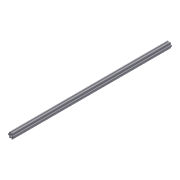
# Autodesk Inventor part: CrossHex 1825
Saved by Autodesk Inventor 2011 (Build 150239000, 239)
## iProperties
Created: 2011-07-24
Part Number: CrossHex 1825
Material: Aluminum-6061
Document SubType Name: Modeling
Designer: Dan Niemitalo
Mass: 103.792 g
Surface Area: 304.789 cm^2
Volume: 38.2997 cm^3
Density: 2.71 g/cm^3
Author: Dan Niemitalo
Autodesk Inventor part; units mm, degrees
ref_plane "YZ Plane" through (0, 0, 0) normal (1, 0, 0) x (0, 1, 0)
ref_plane "XZ Plane" through (0, 0, 0) normal (0, 1, 0) x (-1, 0, 0)
ref_plane "XY Plane" through (0, 0, 0) normal (0, 0, 1) x (1, 0, 0)
sketch "CrossHexProfile" plane through (0, 0, 0) normal (0, 0, 1) x (1, 0, 0)
  arc A0 (1.7598, 0) -> (1.5084, -0.2177) centre (1.7598, -0.254) ccw
  line L0 (1.7598, 0) -> (3.5929, 0)
  arc A1 (3.7028, -0.0635) -> (3.5929, 0) centre (3.5929, -0.127) ccw
  line L1 (3.7028, -0.0635) -> (4.6194, -1.651)
  arc A2 (4.5565, -1.9776) -> (4.6194, -1.651) centre (4.3994, -1.778) ccw
  arc A3 (4.5565, -1.9776) -> (6.0649, -4.5901) centre (5.4993, -3.175) ccw
  arc A4 (-1.5084, -0.2177) -> (1.5084, -0.2177) centre (0, 0) ccw
  arc A5 (-4.5565, -10.7224) -> (-4.6194, -11.049) centre (-4.3994, -10.922) ccw
  arc A6 (-4.5565, -10.7224) -> (-6.0649, -8.1099) centre (-5.4993, -9.525) ccw
  arc A7 (-6.3791, -8.001) -> (-6.0649, -8.1099) centre (-6.1592, -7.874) ccw
  line L2 (-6.3791, -8.001) -> (-7.2957, -6.4135)
  arc A8 (-7.2957, -6.2865) -> (-7.2957, -6.4135) centre (-7.1857, -6.35) ccw
  arc A9 (-6.0649, -4.5901) -> (-6.3791, -4.699) centre (-6.1592, -4.826) ccw
  line L3 (-7.2957, -6.2865) -> (-6.3791, -4.699)
  arc A10 (-1.5084, -0.2177) -> (-1.7598, 0) centre (-1.7598, -0.254) ccw
  line L4 (-3.5929, 0) -> (-1.7598, 0)
  arc A11 (-3.5929, 0) -> (-3.7028, -0.0635) centre (-3.5929, -0.127) ccw
  line L5 (-4.6194, -1.651) -> (-3.7028, -0.0635)
  arc A12 (-4.6194, -1.651) -> (-4.5565, -1.9776) centre (-4.3994, -1.778) ccw
  arc A13 (-6.0649, -4.5901) -> (-4.5565, -1.9776) centre (-5.4993, -3.175) ccw
  line L6 (-3.7028, -12.6365) -> (-4.6194, -11.049)
  circle A14 centre (0, -6.35) radius 2.9337
  arc A15 (-3.7028, -12.6365) -> (-3.5929, -12.7) centre (-3.5929, -12.573) ccw
  line L7 (-1.7598, -12.7) -> (-3.5929, -12.7)
  arc A16 (-1.7598, -12.7) -> (-1.5084, -12.4823) centre (-1.7598, -12.446) ccw
  arc A17 (1.5084, -12.4823) -> (-1.5084, -12.4823) centre (0, -12.7) ccw
  arc A18 (1.5084, -12.4823) -> (1.7598, -12.7) centre (1.7598, -12.446) ccw
  line L8 (3.5929, -12.7) -> (1.7598, -12.7)
  arc A19 (3.5929, -12.7) -> (3.7028, -12.6365) centre (3.5929, -12.573) ccw
  line L9 (4.6194, -11.049) -> (3.7028, -12.6365)
  arc A20 (6.3791, -4.699) -> (6.0649, -4.5901) centre (6.1592, -4.826) ccw
  line L10 (6.3791, -4.699) -> (7.2957, -6.2865)
  arc A21 (7.2957, -6.4135) -> (7.2957, -6.2865) centre (7.1857, -6.35) ccw
  arc A22 (6.0649, -8.1099) -> (6.3791, -8.001) centre (6.1592, -7.874) ccw
  line L11 (7.2957, -6.4135) -> (6.3791, -8.001)
  arc A23 (4.6194, -11.049) -> (4.5565, -10.7224) centre (4.3994, -10.922) ccw
  arc A24 (6.0649, -8.1099) -> (4.5565, -10.7224) centre (5.4993, -9.525) ccw
  point P0 (0, -6.35)
sketch "Sketch1" plane through (0, 0, 0) normal (0, 0, 1) x (1, 0, 0)
  arc A0 (1.7598, 6.35) -> (1.5084, 6.1323) centre (1.7598, 6.096) ccw
  line L0 (1.7598, 6.35) -> (3.5929, 6.35)
  arc A1 (3.7028, 6.2865) -> (3.5929, 6.35) centre (3.5929, 6.223) ccw
  line L1 (3.7028, 6.2865) -> (4.6194, 4.699)
  arc A2 (4.5565, 4.3724) -> (4.6194, 4.699) centre (4.3994, 4.572) ccw
  arc A3 (4.5565, 4.3724) -> (6.0649, 1.7599) centre (5.4993, 3.175) ccw
  arc A4 (-1.5084, 6.1323) -> (1.5084, 6.1323) centre (0, 6.35) ccw
  arc A5 (-4.5565, -4.3724) -> (-4.6194, -4.699) centre (-4.3994, -4.572) ccw
  arc A6 (-4.5565, -4.3724) -> (-6.0649, -1.7599) centre (-5.4993, -3.175) ccw
  arc A7 (-6.3791, -1.651) -> (-6.0649, -1.7599) centre (-6.1592, -1.524) ccw
  line L2 (-6.3791, -1.651) -> (-7.2957, -0.0635)
  arc A8 (-7.2957, 0.0635) -> (-7.2957, -0.0635) centre (-7.1857, 0) ccw
  arc A9 (-6.0649, 1.7599) -> (-6.3791, 1.651) centre (-6.1592, 1.524) ccw
  line L3 (-7.2957, 0.0635) -> (-6.3791, 1.651)
  arc A10 (-1.5084, 6.1323) -> (-1.7598, 6.35) centre (-1.7598, 6.096) ccw
  line L4 (-3.5929, 6.35) -> (-1.7598, 6.35)
  arc A11 (-3.5929, 6.35) -> (-3.7028, 6.2865) centre (-3.5929, 6.223) ccw
  line L5 (-4.6194, 4.699) -> (-3.7028, 6.2865)
  arc A12 (-4.6194, 4.699) -> (-4.5565, 4.3724) centre (-4.3994, 4.572) ccw
  arc A13 (-6.0649, 1.7599) -> (-4.5565, 4.3724) centre (-5.4993, 3.175) ccw
  line L6 (-3.7028, -6.2865) -> (-4.6194, -4.699)
  circle A14 centre (0, 0) radius 2.9337
  arc A15 (-3.7028, -6.2865) -> (-3.5929, -6.35) centre (-3.5929, -6.223) ccw
  line L7 (-1.7598, -6.35) -> (-3.5929, -6.35)
  arc A16 (-1.7598, -6.35) -> (-1.5084, -6.1323) centre (-1.7598, -6.096) ccw
  arc A17 (1.5084, -6.1323) -> (-1.5084, -6.1323) centre (0, -6.35) ccw
  arc A18 (1.5084, -6.1323) -> (1.7598, -6.35) centre (1.7598, -6.096) ccw
  line L8 (3.5929, -6.35) -> (1.7598, -6.35)
  arc A19 (3.5929, -6.35) -> (3.7028, -6.2865) centre (3.5929, -6.223) ccw
  line L9 (4.6194, -4.699) -> (3.7028, -6.2865)
  arc A20 (6.3791, 1.651) -> (6.0649, 1.7599) centre (6.1592, 1.524) ccw
  line L10 (6.3791, 1.651) -> (7.2957, 0.0635)
  arc A21 (7.2957, -0.0635) -> (7.2957, 0.0635) centre (7.1857, 0) ccw
  arc A22 (6.0649, -1.7599) -> (6.3791, -1.651) centre (6.1592, -1.524) ccw
  line L11 (7.2957, -0.0635) -> (6.3791, -1.651)
  arc A23 (4.6194, -4.699) -> (4.5565, -4.3724) centre (4.3994, -4.572) ccw
  arc A24 (6.0649, -1.7599) -> (4.5565, -4.3724) centre (5.4993, -3.175) ccw
  point P0 (0, 0)
  constraints: 1 other
extrude "Extrusion1" add sketch "Sketch1" along normal blind 377.825
body "Solid1"
